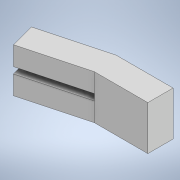
# Autodesk Inventor part: Equerre_gauche
Saved by Autodesk Inventor 2021 (Build 250183000, 183)
## iProperties
Created: 2021-01-15
Part Number: Equerre_gauche
Material: Générique
Document SubType Name: Modeling
Designer: dimercur
Density: 1 g/cm^3
Appearance: Par défaut
Author: dimercur
Autodesk Inventor part; units mm, degrees
ref_plane "YZ Plane" through (0, 0, 0) normal (1, 0, 0) x (0, 1, 0)
ref_plane "XZ Plane" through (0, 0, 0) normal (0, 1, 0) x (-1, 0, 0)
ref_plane "XY Plane" through (0, 0, 0) normal (0, 0, 1) x (1, 0, 0)
sketch "Esquisse1" plane through (0, 0, 0) normal (0, 1, 0) x (-1, 0, 0)
  line L0 (53.1259, 14.235) -> (0, 0)
  line L1 (47.9495, 33.5536) -> (53.1259, 14.235)
  line L2 (-45, 0) -> (-45, 20)
  line L3 (-45, 0) -> (0, 0)
  line L4 (-45, 20) -> (-2.633, 20)
  line L5 (47.9495, 33.5536) -> (-2.633, 20)
  dimension "d1" = 20
  dimension "d4" = 20
  dimension "d7" = 45
  dimension "d9" = 55
  dimension "d11" = 15
  constraints: 12 end point, 2 horizontal, 1 parallel, 1 perpendicular, 1 vertical
  measures "d1" distance of L1.start L0.start
  measures "d4" distance of L2.start L2.end
  measures "d7" distance of L2.start L0.end
  measures "d9" distance of L0.start L0.end
  measures "d11" angle of L0 L3
extrude "Extrusion1" add sketch "Esquisse1" along normal blind 35
sketch "Esquisse3" plane through (2.633, 0, 20) normal (0, 0, 1) x (1, 0, 0)
  line L0 (0, 0) -> (0, 35) projected
  line L1 (-65, 20) -> (0, 20)
  line L2 (0, 20) -> (0, 15)
  line L3 (0, 15) -> (-65, 15)
  line L4 (-65, 15) -> (-65, 20)
  line L5 (-2.633, 35) -> (-55.759, 35) projected
  point P0 (-2.633, 0)
  point P1 (0, 20)
  dimension "d14" = 5
  dimension "d15" = 65
  dimension "d16" = 15
  constraints: 8 end point, 2 parallel, 1 horizontal, 1 perpendicular, 1 point on line
  measures "d14" distance of L3.end L1.start
  measures "d15" distance of L1.start L1.end
  measures "d16" distance between parallel lines of L5 L1
extrude "Extrusion2" cut sketch "Esquisse3" along normal through all both and the other way through all
equation "\"d1\" = d4"
